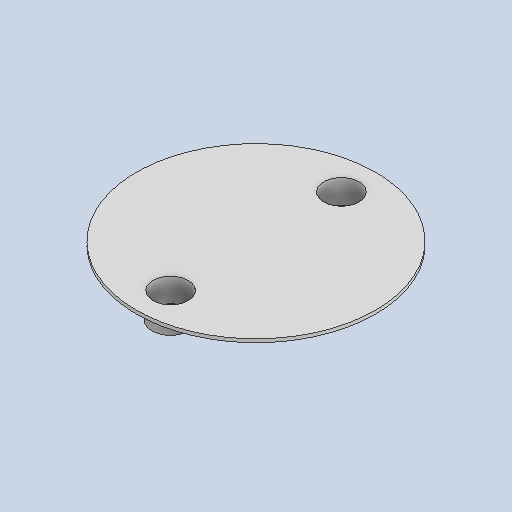
# Autodesk Inventor part: magnet_holder
Saved by Autodesk Inventor 2025 (Build 290162000, 162)
## iProperties
Created: 2025-08-16
Part Number: magnet_holder
Material: Generic
Document SubType Name: Modeling
Designer: Pravoslav
Density: 1 g/cm^3
Appearance: Default
Author: Pravoslav
Autodesk Inventor part; units mm, degrees
ref_plane "YZ Plane" through (0, 0, 0) normal (1, 0, 0) x (0, 1, 0)
ref_plane "XZ Plane" through (0, 0, 0) normal (0, 1, 0) x (-1, 0, 0)
ref_plane "XY Plane" through (0, 0, 0) normal (0, 0, 1) x (1, 0, 0)
sketch "Sketch1" plane through (0, 0, 0) normal (0, 1, 0) x (-1, 0, 0)
  circle A0 centre (0, 0) radius 18
  circle A1 centre (0, 0) radius 19
  dimension "d0" = 36
  dimension "d1" = 38
  constraints: 2 centre point, 2 coincident
  measures "d0" diameter of A0
  measures "d1" diameter of A1
extrude "Extrusion1" add sketch "Sketch1" along normal blind 5
sketch "Sketch2" plane through (0, 5, 0) normal (0, 1, 0) x (1, 0, 0)
  circle A0 centre (0, 0) radius 35
  circle A1 centre (0, 0) radius 19 projected
  circle A2 centre (0, -25) radius 5.15
  circle A3 centre (0, 25) radius 5.15
  dimension "d4" = 16
  dimension "d5" = 10.3
  dimension "d6" = 10.3
  dimension "d7" = 25
  dimension "d8" = 25
  constraints: 3 centre point, 1 coincident
  measures "d4" radial gap between concentric circles of A0 A1
  measures "d5" diameter of A2
  measures "d6" diameter of A3
  measures "d7" distance of A0.centre A2.centre
  measures "d8" distance of A0.centre A3.centre
extrude "Extrusion2" add sketch "Sketch2" along normal blind 1 contours A0 | A1
sketch "Sketch3" plane through (0, 5, 0) normal (0, -1, 0) x (1, 0, 0)
  circle A0 centre (0, 25) radius 5.15
  circle A1 centre (0, -25) radius 5.15
  circle A2 centre (0, -25) radius 5.15 projected
  circle A3 centre (0, 25) radius 5.15 projected
  circle A4 centre (0, 25) radius 5.5
  circle A5 centre (0, -25) radius 5.5
  point P0 (0, 0)
  point P1 (-4.4822, -18.4638)
  point P2 (4.4822, -18.4638)
  point P3 (4.4822, 18.4638)
  point P4 (-4.4822, 18.4638)
  dimension "d11" = 10.3
  dimension "d12" = 10.3
  dimension "d13" = 0
  dimension "d14" = 0
  dimension "d15" = 11
  dimension "d16" = 11
  constraints: 2 centre point, 2 coincident, 6 other
  measures "d15" diameter of A4
  measures "d16" diameter of A5
extrude "Extrusion3" add sketch "Sketch3" along normal blind 6
sketch "Sketch4" plane through (0, -1, 25) normal (0, -1, 0) x (1, 0, 0)
  circle A0 centre (0, 0) radius 5.5
  circle A1 centre (0, -50) radius 5.5
  circle A2 centre (0, -50) radius 5.5 projected
  point P0 (0, -25)
  dimension "d19" = 11
  dimension "d20" = 0
  constraints: 2 centre point
  measures "d19" diameter of A1
  measures "d20" radial gap between concentric circles of A2 A1
extrude "Extrusion4" add sketch "Sketch4" along normal blind 0.5
body "Solid1"
